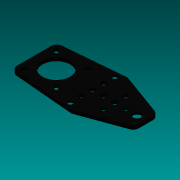
# Autodesk Inventor part: 2020 Slider Motorized
Saved by Autodesk Inventor 2016 (Build 200138000, 138)
## iProperties
Created: 2015-06-04
Part Number: 2020 Slider Motorized
Material: Aluminum 6061
Document SubType Name: Modeling
Designer: Sawaiz Syed
Density: 2.7 g/cm^3
Appearance: Anodized - Black
Author: Sawaiz Syed
Autodesk Inventor part; units mm, degrees
ref_plane "YZ Plane" through (0, 0, 0) normal (1, 0, 0) x (0, 1, 0)
ref_plane "XZ Plane" through (0, 0, 0) normal (0, 1, 0) x (-1, 0, 0)
ref_plane "XY Plane" through (0, 0, 0) normal (0, 0, 1) x (1, 0, 0)
sketch "Sketch1" plane through (0, 0, 0) normal (0, 0, 1) x (1, 0, 0)
  circle A0 centre (80.14, 40.64) radius 3.57 projected
  circle A1 centre (40.14, 40.64) radius 2.5 projected
  circle A2 centre (40.14, 50.64) radius 2.5 projected
  circle A3 centre (40.14, 60.64) radius 2.5 projected
  circle A4 centre (40.14, 30.64) radius 2.5 projected
  circle A5 centre (40.14, 20.64) radius 2.5 projected
  circle A6 centre (7.59, 40.64) radius 12.5 projected
  arc A7 (-4.314, 26.544) -> (-6.506, 28.736) centre (-5.41, 27.64) ccw projected
  line L0 (-6.814, 24.044) -> (-4.314, 26.544) projected
  arc A8 (-9.006, 26.236) -> (-6.814, 24.044) centre (-7.91, 25.14) ccw projected
  line L1 (-6.506, 28.736) -> (-9.006, 26.236) projected
  line L2 (-4.314, 54.736) -> (-6.814, 57.236) projected
  arc A9 (-6.506, 52.544) -> (-4.314, 54.736) centre (-5.41, 53.64) ccw projected
  line L3 (-9.006, 55.044) -> (-6.506, 52.544) projected
  arc A10 (-6.814, 57.236) -> (-9.006, 55.044) centre (-7.91, 56.14) ccw projected
  line L4 (21.994, 57.236) -> (19.494, 54.736) projected
  arc A11 (19.494, 54.736) -> (21.686, 52.544) centre (20.59, 53.64) ccw projected
  line L5 (21.686, 52.544) -> (24.186, 55.044) projected
  arc A12 (24.186, 55.044) -> (21.994, 57.236) centre (23.09, 56.14) ccw projected
  line L6 (24.186, 26.236) -> (21.686, 28.736) projected
  arc A13 (21.686, 28.736) -> (19.494, 26.544) centre (20.59, 27.64) ccw projected
  line L7 (19.494, 26.544) -> (21.994, 24.044) projected
  arc A14 (21.994, 24.044) -> (24.186, 26.236) centre (23.09, 25.14) ccw projected
  circle A15 centre (60.14, 40.64) radius 2.55 projected
  circle A16 centre (60.14, 30.64) radius 2.55 projected
  circle A17 centre (70.14, 40.64) radius 2.5 projected
  circle A18 centre (60.14, 50.64) radius 2.55 projected
  circle A19 centre (50.14, 40.64) radius 2.5 projected
  line L8 (-12.41, 60.64) -> (-12.41, 20.64)
  line L9 (-12.41, 20.64) -> (46.5039, 15.4857)
  line L10 (46.5039, 15.4857) -> (88.14, 30.64)
  line L11 (88.14, 30.64) -> (88.14, 50.64)
  line L12 (88.14, 50.64) -> (46.5039, 65.7943)
  line L13 (46.5039, 65.7943) -> (-12.41, 60.64)
  point P0 (0, 0)
  dimension "d0" = 40
  dimension "d1" = 20
  dimension "d2" = 20
  dimension "d3" = 8
  dimension "d4" = 10
  dimension "d5" = 20
  dimension "d6" = 95
  dimension "d7" = 95
  dimension "d8" = 110
  dimension "d9" = 110
  constraints: 12 end point, 1 parallel, 1 vertical
  measures "d0" distance of L8.start L8.end
  measures "d1" distance of L10.end L11.end
  measures "d2" distance from line of A6.centre L8
  measures "d3" distance from line of L11 A0.centre
  measures "d4" vertical distance of L10.end A0.centre
  measures "d5" horizontal distance of L8.end A6.centre
  measures "d6" angle of L8 L13
  measures "d7" angle of L8 L9
  measures "d8" angle of L12 L11
  measures "d9" angle of L10 L11
extrude "Extrusion1" add sketch "Sketch1" along normal blind 3
fillet "Fillet1" radius 5 6 edges at (-12.41, 20.64, 1.5) (46.5039, 15.4857, 1.5) (-12.41, 60.64, 1.5) (46.5039, 65.7943, 1.5) (88.14, 50.64, 1.5) (88.14, 30.64, 1.5)
sketch "Sketch2" plane through (0, 0, 0) normal (0, 0, -1) x (-1, 0, 0)
  circle A0 centre (-40.14, 20.64) radius 2.5 projected
  circle A1 centre (-80.14, 40.64) radius 3.57 projected
  circle A2 centre (-40.14, 60.64) radius 2.5 projected
  point P0 (0, 0)
  constraints: 2 coincident
hole "Hole1" at (40.14, 20.64, 0) at (40.14, 60.64, 0) direction (0, 0, 1) diameter 8.1 depth 1
sketch "Sketch3" plane through (0, 0, 0) normal (0, 0, -1) x (-1, 0, 0)
  circle A0 centre (-80.14, 40.64) radius 3.57 projected
  point P0 (0, 0)
  constraints: 1 coincident
hole "Hole2" at (80.14, 40.64, 0) direction (0, 0, 1) diameter 14 depth 1
equation "\"d7\" = d6"
body "Solid1"
